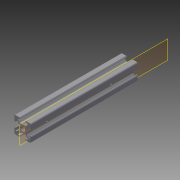
# Autodesk Inventor part: custom bosch 5in
Saved by Autodesk Inventor 2013 (Build 170138000, 138)
## iProperties
Created: 2013-12-23
Part Number: custom bosch 5in
Material: Generic
Document SubType Name: Modeling
Designer: kahohbein
Density: 1 g/cm^3
Author: kahohbein
Autodesk Inventor part; units mm, degrees
ref_plane "YZ Plane" through (0, 0, 0) normal (1, 0, 0) x (0, 1, 0)
ref_plane "XZ Plane" through (0, 0, 0) normal (0, 1, 0) x (-1, 0, 0)
ref_plane "XY Plane" through (0, 0, 0) normal (0, 0, 1) x (1, 0, 0)
sketch "20x20" plane through (0, 0, 0) normal (0, 0, 1) x (1, 0, 0)
  arc A0 (0, 20) -> (-1.5, 18.5) centre (0, 18.5) ccw
  line L0 (-1.5, 18.5) -> (-1.5, 13.75)
  arc A1 (-1.5, 13.75) -> (-1.3, 13.55) centre (-1.3, 13.75) ccw
  line L1 (-1.3, 13.55) -> (-1.2, 13.55)
  arc A2 (-1, 13.35) -> (-1.2, 13.55) centre (-1.2, 13.35) ccw
  line L2 (-1, 13.35) -> (-1, 13.2)
  arc A3 (-1, 13.2) -> (-0.8, 13) centre (-0.8, 13.2) ccw
  line L3 (-0.8, 13) -> (-0.5, 13)
  arc A4 (-0.5, 13) -> (0, 13.5) centre (-0.5, 13.5) ccw
  line L4 (0, 13.5) -> (0, 15.5)
  arc A5 (0.5, 16) -> (0, 15.5) centre (0.5, 15.5) ccw
  line L5 (0.5, 16) -> (1.2322, 16)
  arc A6 (1.5858, 15.8536) -> (1.2322, 16) centre (1.2322, 15.5) ccw
  line L6 (1.5858, 15.8536) -> (3.8536, 13.5858)
  arc A7 (4, 13.2322) -> (3.8536, 13.5858) centre (3.5, 13.2322) ccw
  line L7 (4, 13.2322) -> (4, 10.9536)
  arc A8 (4, 10.9536) -> (4.0268, 10.8536) centre (4.2, 10.9536) ccw
  line L8 (4.0268, 10.8536) -> (4.4619, 10.1)
  arc A9 (4.4619, 9.9) -> (4.4619, 10.1) centre (4.2887, 10) ccw
  line L9 (4.4619, 9.9) -> (4.0268, 9.1464)
  arc A10 (4.0268, 9.1464) -> (4, 9.0464) centre (4.2, 9.0464) ccw
  line L10 (4, 9.0464) -> (4, 6.7678)
  arc A11 (3.8536, 6.4142) -> (4, 6.7678) centre (3.5, 6.7678) ccw
  line L11 (3.8536, 6.4142) -> (1.5858, 4.1464)
  arc A12 (1.2322, 4) -> (1.5858, 4.1464) centre (1.2322, 4.5) ccw
  line L12 (1.2322, 4) -> (0.5, 4)
  arc A13 (0, 4.5) -> (0.5, 4) centre (0.5, 4.5) ccw
  line L13 (0, 4.5) -> (0, 6.5)
  arc A14 (0, 6.5) -> (-0.5, 7) centre (-0.5, 6.5) ccw
  line L14 (-0.5, 7) -> (-0.8, 7)
  arc A15 (-0.8, 7) -> (-1, 6.8) centre (-0.8, 6.8) ccw
  line L15 (-1, 6.8) -> (-1, 6.65)
  arc A16 (-1.2, 6.45) -> (-1, 6.65) centre (-1.2, 6.65) ccw
  line L16 (-1.2, 6.45) -> (-1.3, 6.45)
  arc A17 (-1.3, 6.45) -> (-1.5, 6.25) centre (-1.3, 6.25) ccw
  line L17 (-1.5, 6.25) -> (-1.5, 1.5)
  arc A18 (-1.5, 1.5) -> (0, 0) centre (0, 1.5) ccw
  line L18 (0, 0) -> (4.75, 0)
  arc A19 (4.75, 0) -> (4.95, 0.2) centre (4.75, 0.2) ccw
  line L19 (4.95, 0.2) -> (4.95, 0.3)
  arc A20 (5.15, 0.5) -> (4.95, 0.3) centre (5.15, 0.3) ccw
  line L20 (5.15, 0.5) -> (5.3, 0.5)
  arc A21 (5.3, 0.5) -> (5.5, 0.7) centre (5.3, 0.7) ccw
  line L21 (5.5, 0.7) -> (5.5, 1)
  arc A22 (5.5, 1) -> (5, 1.5) centre (5, 1) ccw
  line L22 (5, 1.5) -> (3, 1.5)
  arc A23 (2.5, 2) -> (3, 1.5) centre (3, 2) ccw
  line L23 (2.5, 2) -> (2.5, 2.7322)
  arc A24 (2.6464, 3.0858) -> (2.5, 2.7322) centre (3, 2.7322) ccw
  line L24 (2.6464, 3.0858) -> (4.9142, 5.3536)
  arc A25 (5.2678, 5.5) -> (4.9142, 5.3536) centre (5.2678, 5) ccw
  line L25 (5.2678, 5.5) -> (7.5464, 5.5)
  arc A26 (7.5464, 5.5) -> (7.6464, 5.5268) centre (7.5464, 5.7) ccw
  line L26 (7.6464, 5.5268) -> (8.4, 5.9619)
  arc A27 (8.6, 5.9619) -> (8.4, 5.9619) centre (8.5, 5.7887) ccw
  line L27 (8.6, 5.9619) -> (9.3536, 5.5268)
  arc A28 (9.3536, 5.5268) -> (9.4536, 5.5) centre (9.4536, 5.7) ccw
  line L28 (9.4536, 5.5) -> (11.7322, 5.5)
  arc A29 (12.0858, 5.3536) -> (11.7322, 5.5) centre (11.7322, 5) ccw
  line L29 (12.0858, 5.3536) -> (14.3536, 3.0858)
  arc A30 (14.5, 2.7322) -> (14.3536, 3.0858) centre (14, 2.7322) ccw
  line L30 (14.5, 2.7322) -> (14.5, 2)
  arc A31 (14, 1.5) -> (14.5, 2) centre (14, 2) ccw
  line L31 (14, 1.5) -> (12, 1.5)
  arc A32 (12, 1.5) -> (11.5, 1) centre (12, 1) ccw
  line L32 (11.5, 1) -> (11.5, 0.7)
  arc A33 (11.5, 0.7) -> (11.7, 0.5) centre (11.7, 0.7) ccw
  line L33 (11.7, 0.5) -> (11.85, 0.5)
  arc A34 (12.05, 0.3) -> (11.85, 0.5) centre (11.85, 0.3) ccw
  line L34 (12.05, 0.3) -> (12.05, 0.2)
  arc A35 (12.05, 0.2) -> (12.25, 0) centre (12.25, 0.2) ccw
  line L35 (12.25, 0) -> (17, 0)
  arc A36 (17, 0) -> (18.5, 1.5) centre (17, 1.5) ccw
  line L36 (18.5, 1.5) -> (18.5, 6.25)
  arc A37 (18.5, 6.25) -> (18.3, 6.45) centre (18.3, 6.25) ccw
  line L37 (18.3, 6.45) -> (18.2, 6.45)
  arc A38 (18, 6.65) -> (18.2, 6.45) centre (18.2, 6.65) ccw
  line L38 (18, 6.65) -> (18, 6.8)
  arc A39 (18, 6.8) -> (17.8, 7) centre (17.8, 6.8) ccw
  line L39 (17.8, 7) -> (17.5, 7)
  arc A40 (17.5, 7) -> (17, 6.5) centre (17.5, 6.5) ccw
  line L40 (17, 6.5) -> (17, 4.5)
  arc A41 (16.5, 4) -> (17, 4.5) centre (16.5, 4.5) ccw
  line L41 (16.5, 4) -> (15.7678, 4)
  arc A42 (15.4142, 4.1464) -> (15.7678, 4) centre (15.7678, 4.5) ccw
  line L42 (15.4142, 4.1464) -> (13.1464, 6.4142)
  arc A43 (13, 6.7678) -> (13.1464, 6.4142) centre (13.5, 6.7678) ccw
  line L43 (13, 6.7678) -> (13, 9.0464)
  arc A44 (13, 9.0464) -> (12.9732, 9.1464) centre (12.8, 9.0464) ccw
  line L44 (12.9732, 9.1464) -> (12.5381, 9.9)
  arc A45 (12.5381, 10.1) -> (12.5381, 9.9) centre (12.7113, 10) ccw
  line L45 (12.5381, 10.1) -> (12.9732, 10.8536)
  arc A46 (12.9732, 10.8536) -> (13, 10.9536) centre (12.8, 10.9536) ccw
  line L46 (13, 10.9536) -> (13, 13.2322)
  arc A47 (13.1464, 13.5858) -> (13, 13.2322) centre (13.5, 13.2322) ccw
  line L47 (13.1464, 13.5858) -> (15.4142, 15.8536)
  arc A48 (15.7678, 16) -> (15.4142, 15.8536) centre (15.7678, 15.5) ccw
  line L48 (15.7678, 16) -> (16.5, 16)
  arc A49 (17, 15.5) -> (16.5, 16) centre (16.5, 15.5) ccw
  line L49 (17, 15.5) -> (17, 13.5)
  arc A50 (17, 13.5) -> (17.5, 13) centre (17.5, 13.5) ccw
  line L50 (17.5, 13) -> (17.8, 13)
  arc A51 (17.8, 13) -> (18, 13.2) centre (17.8, 13.2) ccw
  line L51 (18, 13.2) -> (18, 13.35)
  arc A52 (18.2, 13.55) -> (18, 13.35) centre (18.2, 13.35) ccw
  line L52 (18.2, 13.55) -> (18.3, 13.55)
  arc A53 (18.3, 13.55) -> (18.5, 13.75) centre (18.3, 13.75) ccw
  line L53 (18.5, 13.75) -> (18.5, 18.5)
  arc A54 (18.5, 18.5) -> (17, 20) centre (17, 18.5) ccw
  line L54 (17, 20) -> (12.25, 20)
  arc A55 (12.25, 20) -> (12.05, 19.8) centre (12.25, 19.8) ccw
  line L55 (12.05, 19.8) -> (12.05, 19.7)
  arc A56 (11.85, 19.5) -> (12.05, 19.7) centre (11.85, 19.7) ccw
  line L56 (11.85, 19.5) -> (11.7, 19.5)
  arc A57 (11.7, 19.5) -> (11.5, 19.3) centre (11.7, 19.3) ccw
  line L57 (11.5, 19.3) -> (11.5, 19)
  arc A58 (11.5, 19) -> (12, 18.5) centre (12, 19) ccw
  line L58 (12, 18.5) -> (14, 18.5)
  arc A59 (14.5, 18) -> (14, 18.5) centre (14, 18) ccw
  line L59 (14.5, 18) -> (14.5, 17.2678)
  arc A60 (14.3536, 16.9142) -> (14.5, 17.2678) centre (14, 17.2678) ccw
  line L60 (14.3536, 16.9142) -> (12.0858, 14.6464)
  arc A61 (11.7322, 14.5) -> (12.0858, 14.6464) centre (11.7322, 15) ccw
  line L61 (11.7322, 14.5) -> (9.4536, 14.5)
  arc A62 (9.4536, 14.5) -> (9.3536, 14.4732) centre (9.4536, 14.3) ccw
  line L62 (9.3536, 14.4732) -> (8.6, 14.0381)
  arc A63 (8.4, 14.0381) -> (8.6, 14.0381) centre (8.5, 14.2113) ccw
  line L63 (8.4, 14.0381) -> (7.6464, 14.4732)
  arc A64 (7.6464, 14.4732) -> (7.5464, 14.5) centre (7.5464, 14.3) ccw
  line L64 (7.5464, 14.5) -> (5.2678, 14.5)
  arc A65 (4.9142, 14.6464) -> (5.2678, 14.5) centre (5.2678, 15) ccw
  line L65 (4.9142, 14.6464) -> (2.6464, 16.9142)
  arc A66 (2.5, 17.2678) -> (2.6464, 16.9142) centre (3, 17.2678) ccw
  line L66 (2.5, 17.2678) -> (2.5, 18)
  arc A67 (3, 18.5) -> (2.5, 18) centre (3, 18) ccw
  line L67 (3, 18.5) -> (5, 18.5)
  arc A68 (5, 18.5) -> (5.5, 19) centre (5, 19) ccw
  line L68 (5.5, 19) -> (5.5, 19.3)
  arc A69 (5.5, 19.3) -> (5.3, 19.5) centre (5.3, 19.3) ccw
  line L69 (5.3, 19.5) -> (5.15, 19.5)
  arc A70 (4.95, 19.7) -> (5.15, 19.5) centre (5.15, 19.7) ccw
  line L70 (4.95, 19.7) -> (4.95, 19.8)
  arc A71 (4.95, 19.8) -> (4.75, 20) centre (4.75, 19.8) ccw
  line L71 (4.75, 20) -> (0, 20)
  arc A72 (6.5861, 12.9896) -> (5.5078, 11.9099) centre (8.5, 10) ccw
  line L72 (7.2418, 12.4453) -> (6.5861, 12.9896)
  arc A73 (9.7582, 12.4453) -> (7.2418, 12.4453) centre (8.5, 10) ccw
  line L73 (10.4139, 12.9896) -> (9.7582, 12.4453)
  arc A74 (11.4922, 11.9099) -> (10.4139, 12.9896) centre (8.5, 10) ccw
  line L74 (10.9453, 11.2582) -> (11.4922, 11.9099)
  arc A75 (10.9453, 8.7418) -> (10.9453, 11.2582) centre (8.5, 10) ccw
  line L75 (11.4922, 8.0901) -> (10.9453, 8.7418)
  arc A76 (10.4139, 7.0104) -> (11.4922, 8.0901) centre (8.5, 10) ccw
  line L76 (9.7582, 7.5547) -> (10.4139, 7.0104)
  arc A77 (7.2418, 7.5547) -> (9.7582, 7.5547) centre (8.5, 10) ccw
  line L77 (6.5861, 7.0104) -> (7.2418, 7.5547)
  arc A78 (5.5078, 8.0901) -> (6.5861, 7.0104) centre (8.5, 10) ccw
  line L78 (6.0547, 8.7418) -> (5.5078, 8.0901)
  arc A79 (6.0547, 11.2582) -> (6.0547, 8.7418) centre (8.5, 10) ccw
  line L79 (5.5078, 11.9099) -> (6.0547, 11.2582)
  point P0 (8.5, 10)
sketch "Sketch1" plane through (0, 0, 0) normal (0, 0, 1) x (1, 0, 0)
  arc A0 (-8.5, 10) -> (-10, 8.5) centre (-8.5, 8.5) ccw
  line L0 (-10, 8.5) -> (-10, 3.75)
  arc A1 (-10, 3.75) -> (-9.8, 3.55) centre (-9.8, 3.75) ccw
  line L1 (-9.8, 3.55) -> (-9.7, 3.55)
  arc A2 (-9.5, 3.35) -> (-9.7, 3.55) centre (-9.7, 3.35) ccw
  line L2 (-9.5, 3.35) -> (-9.5, 3.2)
  arc A3 (-9.5, 3.2) -> (-9.3, 3) centre (-9.3, 3.2) ccw
  line L3 (-9.3, 3) -> (-9, 3)
  arc A4 (-9, 3) -> (-8.5, 3.5) centre (-9, 3.5) ccw
  line L4 (-8.5, 3.5) -> (-8.5, 5.5)
  arc A5 (-8, 6) -> (-8.5, 5.5) centre (-8, 5.5) ccw
  line L5 (-8, 6) -> (-7.2678, 6)
  arc A6 (-6.9142, 5.8536) -> (-7.2678, 6) centre (-7.2678, 5.5) ccw
  line L6 (-6.9142, 5.8536) -> (-4.6464, 3.5858)
  arc A7 (-4.5, 3.2322) -> (-4.6464, 3.5858) centre (-5, 3.2322) ccw
  line L7 (-4.5, 3.2322) -> (-4.5, 0.9536)
  arc A8 (-4.5, 0.9536) -> (-4.4732, 0.8536) centre (-4.3, 0.9536) ccw
  line L8 (-4.4732, 0.8536) -> (-4.0381, 0.1)
  arc A9 (-4.0381, -0.1) -> (-4.0381, 0.1) centre (-4.2113, 0) ccw
  line L9 (-4.0381, -0.1) -> (-4.4732, -0.8536)
  arc A10 (-4.4732, -0.8536) -> (-4.5, -0.9536) centre (-4.3, -0.9536) ccw
  line L10 (-4.5, -0.9536) -> (-4.5, -3.2322)
  arc A11 (-4.6464, -3.5858) -> (-4.5, -3.2322) centre (-5, -3.2322) ccw
  line L11 (-4.6464, -3.5858) -> (-6.9142, -5.8536)
  arc A12 (-7.2678, -6) -> (-6.9142, -5.8536) centre (-7.2678, -5.5) ccw
  line L12 (-7.2678, -6) -> (-8, -6)
  arc A13 (-8.5, -5.5) -> (-8, -6) centre (-8, -5.5) ccw
  line L13 (-8.5, -5.5) -> (-8.5, -3.5)
  arc A14 (-8.5, -3.5) -> (-9, -3) centre (-9, -3.5) ccw
  line L14 (-9, -3) -> (-9.3, -3)
  arc A15 (-9.3, -3) -> (-9.5, -3.2) centre (-9.3, -3.2) ccw
  line L15 (-9.5, -3.2) -> (-9.5, -3.35)
  arc A16 (-9.7, -3.55) -> (-9.5, -3.35) centre (-9.7, -3.35) ccw
  line L16 (-9.7, -3.55) -> (-9.8, -3.55)
  arc A17 (-9.8, -3.55) -> (-10, -3.75) centre (-9.8, -3.75) ccw
  line L17 (-10, -3.75) -> (-10, -8.5)
  arc A18 (-10, -8.5) -> (-8.5, -10) centre (-8.5, -8.5) ccw
  line L18 (-8.5, -10) -> (-3.75, -10)
  arc A19 (-3.75, -10) -> (-3.55, -9.8) centre (-3.75, -9.8) ccw
  line L19 (-3.55, -9.8) -> (-3.55, -9.7)
  arc A20 (-3.35, -9.5) -> (-3.55, -9.7) centre (-3.35, -9.7) ccw
  line L20 (-3.35, -9.5) -> (-3.2, -9.5)
  arc A21 (-3.2, -9.5) -> (-3, -9.3) centre (-3.2, -9.3) ccw
  line L21 (-3, -9.3) -> (-3, -9)
  arc A22 (-3, -9) -> (-3.5, -8.5) centre (-3.5, -9) ccw
  line L22 (-3.5, -8.5) -> (-5.5, -8.5)
  arc A23 (-6, -8) -> (-5.5, -8.5) centre (-5.5, -8) ccw
  line L23 (-6, -8) -> (-6, -7.2678)
  arc A24 (-5.8536, -6.9142) -> (-6, -7.2678) centre (-5.5, -7.2678) ccw
  line L24 (-5.8536, -6.9142) -> (-3.5858, -4.6464)
  arc A25 (-3.2322, -4.5) -> (-3.5858, -4.6464) centre (-3.2322, -5) ccw
  line L25 (-3.2322, -4.5) -> (-0.9536, -4.5)
  arc A26 (-0.9536, -4.5) -> (-0.8536, -4.4732) centre (-0.9536, -4.3) ccw
  line L26 (-0.8536, -4.4732) -> (-0.1, -4.0381)
  arc A27 (0.1, -4.0381) -> (-0.1, -4.0381) centre (0, -4.2113) ccw
  line L27 (0.1, -4.0381) -> (0.8536, -4.4732)
  arc A28 (0.8536, -4.4732) -> (0.9536, -4.5) centre (0.9536, -4.3) ccw
  line L28 (0.9536, -4.5) -> (3.2322, -4.5)
  arc A29 (3.5858, -4.6464) -> (3.2322, -4.5) centre (3.2322, -5) ccw
  line L29 (3.5858, -4.6464) -> (5.8536, -6.9142)
  arc A30 (6, -7.2678) -> (5.8536, -6.9142) centre (5.5, -7.2678) ccw
  line L30 (6, -7.2678) -> (6, -8)
  arc A31 (5.5, -8.5) -> (6, -8) centre (5.5, -8) ccw
  line L31 (5.5, -8.5) -> (3.5, -8.5)
  arc A32 (3.5, -8.5) -> (3, -9) centre (3.5, -9) ccw
  line L32 (3, -9) -> (3, -9.3)
  arc A33 (3, -9.3) -> (3.2, -9.5) centre (3.2, -9.3) ccw
  line L33 (3.2, -9.5) -> (3.35, -9.5)
  arc A34 (3.55, -9.7) -> (3.35, -9.5) centre (3.35, -9.7) ccw
  line L34 (3.55, -9.7) -> (3.55, -9.8)
  arc A35 (3.55, -9.8) -> (3.75, -10) centre (3.75, -9.8) ccw
  line L35 (3.75, -10) -> (8.5, -10)
  arc A36 (8.5, -10) -> (10, -8.5) centre (8.5, -8.5) ccw
  line L36 (10, -8.5) -> (10, -3.75)
  arc A37 (10, -3.75) -> (9.8, -3.55) centre (9.8, -3.75) ccw
  line L37 (9.8, -3.55) -> (9.7, -3.55)
  arc A38 (9.5, -3.35) -> (9.7, -3.55) centre (9.7, -3.35) ccw
  line L38 (9.5, -3.35) -> (9.5, -3.2)
  arc A39 (9.5, -3.2) -> (9.3, -3) centre (9.3, -3.2) ccw
  line L39 (9.3, -3) -> (9, -3)
  arc A40 (9, -3) -> (8.5, -3.5) centre (9, -3.5) ccw
  line L40 (8.5, -3.5) -> (8.5, -5.5)
  arc A41 (8, -6) -> (8.5, -5.5) centre (8, -5.5) ccw
  line L41 (8, -6) -> (7.2678, -6)
  arc A42 (6.9142, -5.8536) -> (7.2678, -6) centre (7.2678, -5.5) ccw
  line L42 (6.9142, -5.8536) -> (4.6464, -3.5858)
  arc A43 (4.5, -3.2322) -> (4.6464, -3.5858) centre (5, -3.2322) ccw
  line L43 (4.5, -3.2322) -> (4.5, -0.9536)
  arc A44 (4.5, -0.9536) -> (4.4732, -0.8536) centre (4.3, -0.9536) ccw
  line L44 (4.4732, -0.8536) -> (4.0381, -0.1)
  arc A45 (4.0381, 0.1) -> (4.0381, -0.1) centre (4.2113, 0) ccw
  line L45 (4.0381, 0.1) -> (4.4732, 0.8536)
  arc A46 (4.4732, 0.8536) -> (4.5, 0.9536) centre (4.3, 0.9536) ccw
  line L46 (4.5, 0.9536) -> (4.5, 3.2322)
  arc A47 (4.6464, 3.5858) -> (4.5, 3.2322) centre (5, 3.2322) ccw
  line L47 (4.6464, 3.5858) -> (6.9142, 5.8536)
  arc A48 (7.2678, 6) -> (6.9142, 5.8536) centre (7.2678, 5.5) ccw
  line L48 (7.2678, 6) -> (8, 6)
  arc A49 (8.5, 5.5) -> (8, 6) centre (8, 5.5) ccw
  line L49 (8.5, 5.5) -> (8.5, 3.5)
  arc A50 (8.5, 3.5) -> (9, 3) centre (9, 3.5) ccw
  line L50 (9, 3) -> (9.3, 3)
  arc A51 (9.3, 3) -> (9.5, 3.2) centre (9.3, 3.2) ccw
  line L51 (9.5, 3.2) -> (9.5, 3.35)
  arc A52 (9.7, 3.55) -> (9.5, 3.35) centre (9.7, 3.35) ccw
  line L52 (9.7, 3.55) -> (9.8, 3.55)
  arc A53 (9.8, 3.55) -> (10, 3.75) centre (9.8, 3.75) ccw
  line L53 (10, 3.75) -> (10, 8.5)
  arc A54 (10, 8.5) -> (8.5, 10) centre (8.5, 8.5) ccw
  line L54 (8.5, 10) -> (3.75, 10)
  arc A55 (3.75, 10) -> (3.55, 9.8) centre (3.75, 9.8) ccw
  line L55 (3.55, 9.8) -> (3.55, 9.7)
  arc A56 (3.35, 9.5) -> (3.55, 9.7) centre (3.35, 9.7) ccw
  line L56 (3.35, 9.5) -> (3.2, 9.5)
  arc A57 (3.2, 9.5) -> (3, 9.3) centre (3.2, 9.3) ccw
  line L57 (3, 9.3) -> (3, 9)
  arc A58 (3, 9) -> (3.5, 8.5) centre (3.5, 9) ccw
  line L58 (3.5, 8.5) -> (5.5, 8.5)
  arc A59 (6, 8) -> (5.5, 8.5) centre (5.5, 8) ccw
  line L59 (6, 8) -> (6, 7.2678)
  arc A60 (5.8536, 6.9142) -> (6, 7.2678) centre (5.5, 7.2678) ccw
  line L60 (5.8536, 6.9142) -> (3.5858, 4.6464)
  arc A61 (3.2322, 4.5) -> (3.5858, 4.6464) centre (3.2322, 5) ccw
  line L61 (3.2322, 4.5) -> (0.9536, 4.5)
  arc A62 (0.9536, 4.5) -> (0.8536, 4.4732) centre (0.9536, 4.3) ccw
  line L62 (0.8536, 4.4732) -> (0.1, 4.0381)
  arc A63 (-0.1, 4.0381) -> (0.1, 4.0381) centre (0, 4.2113) ccw
  line L63 (-0.1, 4.0381) -> (-0.8536, 4.4732)
  arc A64 (-0.8536, 4.4732) -> (-0.9536, 4.5) centre (-0.9536, 4.3) ccw
  line L64 (-0.9536, 4.5) -> (-3.2322, 4.5)
  arc A65 (-3.5858, 4.6464) -> (-3.2322, 4.5) centre (-3.2322, 5) ccw
  line L65 (-3.5858, 4.6464) -> (-5.8536, 6.9142)
  arc A66 (-6, 7.2678) -> (-5.8536, 6.9142) centre (-5.5, 7.2678) ccw
  line L66 (-6, 7.2678) -> (-6, 8)
  arc A67 (-5.5, 8.5) -> (-6, 8) centre (-5.5, 8) ccw
  line L67 (-5.5, 8.5) -> (-3.5, 8.5)
  arc A68 (-3.5, 8.5) -> (-3, 9) centre (-3.5, 9) ccw
  line L68 (-3, 9) -> (-3, 9.3)
  arc A69 (-3, 9.3) -> (-3.2, 9.5) centre (-3.2, 9.3) ccw
  line L69 (-3.2, 9.5) -> (-3.35, 9.5)
  arc A70 (-3.55, 9.7) -> (-3.35, 9.5) centre (-3.35, 9.7) ccw
  line L70 (-3.55, 9.7) -> (-3.55, 9.8)
  arc A71 (-3.55, 9.8) -> (-3.75, 10) centre (-3.75, 9.8) ccw
  line L71 (-3.75, 10) -> (-8.5, 10)
  arc A72 (-1.9139, 2.9896) -> (-2.9922, 1.9099) centre (0, 0) ccw
  line L72 (-1.2582, 2.4453) -> (-1.9139, 2.9896)
  arc A73 (1.2582, 2.4453) -> (-1.2582, 2.4453) centre (0, 0) ccw
  line L73 (1.9139, 2.9896) -> (1.2582, 2.4453)
  arc A74 (2.9922, 1.9099) -> (1.9139, 2.9896) centre (0, 0) ccw
  line L74 (2.4453, 1.2582) -> (2.9922, 1.9099)
  arc A75 (2.4453, -1.2582) -> (2.4453, 1.2582) centre (0, 0) ccw
  line L75 (2.9922, -1.9099) -> (2.4453, -1.2582)
  arc A76 (1.9139, -2.9896) -> (2.9922, -1.9099) centre (0, 0) ccw
  line L76 (1.2582, -2.4453) -> (1.9139, -2.9896)
  arc A77 (-1.2582, -2.4453) -> (1.2582, -2.4453) centre (0, 0) ccw
  line L77 (-1.9139, -2.9896) -> (-1.2582, -2.4453)
  arc A78 (-2.9922, -1.9099) -> (-1.9139, -2.9896) centre (0, 0) ccw
  line L78 (-2.4453, -1.2582) -> (-2.9922, -1.9099)
  arc A79 (-2.4453, 1.2582) -> (-2.4453, -1.2582) centre (0, 0) ccw
  line L79 (-2.9922, 1.9099) -> (-2.4453, 1.2582)
  constraints: 1 other
extrude "Extrusion1" add sketch "Sketch1" along normal blind 127
ref_plane "Work Plane1" through (4.5, 0.9536, 127) normal (1, 0, 0) x (0, 0, -1)
sketch "Sketch2" plane through (4.5, 0.9536, 127) normal (1, 0, 0) x (0, 0, -1)
  circle A0 centre (24.2388, -0.9536) radius 2.54
  circle A1 centre (100.4388, -0.9536) radius 2.54
  line L0 (24.2388, -0.9536) -> (100.4388, -0.9536)
  point P0 (127, -0.9536)
  dimension "d2" = 5.08
  dimension "d3" = 5.08
  dimension "d4" = 76.2
  constraints: 2 centre point, 2 end point, 1 horizontal
  measures "d2" diameter of A0
  measures "d3" diameter of A1
  measures "d4" distance of L0.start L0.end
extrude "Extrusion2" cut sketch "Sketch2" against normal blind 160.3375
body "Solid1"
